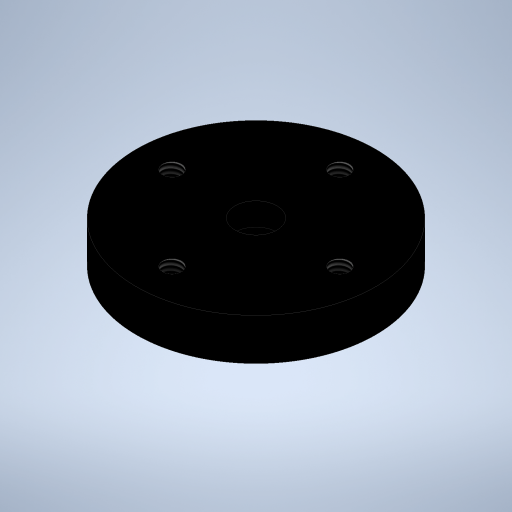
# Autodesk Inventor part: Top Horn Metal
Saved by Autodesk Inventor 2024.1 (Build 281209000, 209)
## iProperties
Created: 2022-09-18
Part Number: Top Horn Metal
Material: 일반
Document SubType Name: Modeling
Designer: 박동준
Density: 1 g/cm^3
Appearance: 기본값
품번: 8
Author: 박동준
Autodesk Inventor part; units mm, degrees
ref_plane "YZ Plane" through (0, 0, 0) normal (1, 0, 0) x (0, 1, 0)
ref_plane "XZ Plane" through (0, 0, 0) normal (0, 1, 0) x (-1, 0, 0)
ref_plane "XY Plane" through (0, 0, 0) normal (0, 0, 1) x (1, 0, 0)
sketch "스케치1" plane through (0, 0, 0) normal (0, 0, 1) x (1, 0, 0)
  line L0 (0, 3.2752) -> (0, -3.2752)
  line L1 (1.75, 3.48) -> (1.75, 1.58)
  line L2 (1.75, 1.58) -> (2.925, 1.58)
  line L3 (2.925, 1.58) -> (2.925, -2.02)
  line L4 (2.925, -2.02) -> (4.5, -2.02)
  line L5 (4.5, -2.02) -> (4.5, 0)
  line L6 (4.5, 0) -> (9.96, 0)
  line L7 (9.96, 0) -> (9.96, 3.48)
  line L8 (9.96, 3.48) -> (1.75, 3.48)
  point P0 (0, 0)
  point P1 (0, 0)
  dimension "d1" = 1.75
  dimension "d2" = 2.925
  dimension "d4" = 3.48
  dimension "d6" = 4.5
  dimension "d7" = 9.96
  dimension "d8" = 1.9
  dimension "d22" = 5.5
  constraints: 18 end point, 4 perpendicular, 2 midpoint, 2 vertical, 1 coincident, 1 horizontal, 1 horizontal alignment, 1 parallel
  measures "d1" distance between parallel lines of L1 L0
  measures "d2" distance between parallel lines of L3 L0
  measures "d4" distance of L7.end L6.end
  measures "d6" distance between parallel lines of L0 L5
  measures "d7" distance between parallel lines of L7 L0
  measures "d8" distance of L1.start L1.end
  measures "d22" distance between parallel lines of L8 L4
revolve "회전1" add sketch "스케치1" angle 360 about axis through (0, 3.2752, 0) along (0, -1, 0)
sketch "Sketch3" plane through (0, 3.48, 0) normal (0, 1, 0) x (1, 0, 0)
  point P0 (0, 0)
  point P1 (7, 0)
  point P2 (0, 7)
  point P3 (-7, 0)
  point P4 (0, -7)
  dimension "d23" = 7
  dimension "d26" = 360
  constraints: 1 horizontal alignment, 5 other
  measures "d23" distance of point (7, 0) point (0, 0)
hole "Hole2" at (7, 3.48, 0) at (0, 3.48, -7) at (-7, 3.48, 0) at (0, 3.48, 7) direction (0, -1, 0) diameter 1.567 end through all thread size "M2x0.4" class "6H" standard "ISO Metric profile"
